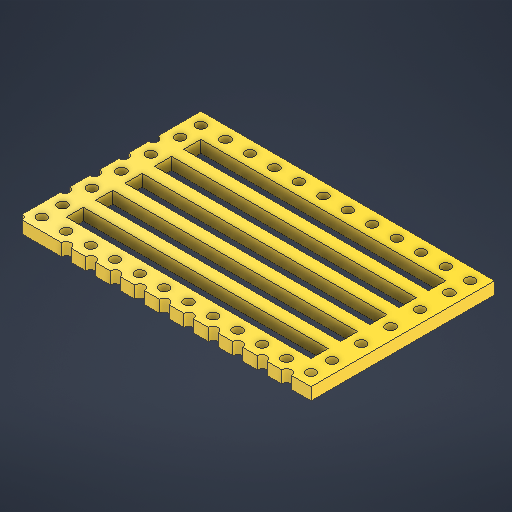
# Autodesk Inventor part: placa_galbena
Saved by Autodesk Inventor 2026.1 (Build 301233000, 233)
## iProperties
Created: 2025-09-04
Part Number: placa_galbena
Material: Generic
Document SubType Name: Modeling
Designer: emanuel
Density: 1 g/cm^3
Appearance: Default
Author: emanuel
Autodesk Inventor part; units mm, degrees
ref_plane "YZ Plane" through (0, 0, 0) normal (1, 0, 0) x (0, 1, 0)
ref_plane "XZ Plane" through (0, 0, 0) normal (0, 1, 0) x (-1, 0, 0)
ref_plane "XY Plane" through (0, 0, 0) normal (0, 0, 1) x (1, 0, 0)
sketch "Sketch1" plane through (0, 0, 0) normal (0, 1, 0) x (-1, 0, 0)
  line L0 (0, 0) -> (60, 0)
  line L1 (60, 0) -> (60, -37.5)
  line L2 (60, -37.5) -> (0, -37.5)
  line L3 (0, -37.5) -> (0, 0)
  line L4 (60, 0) -> (55, 0)
  line L5 (55, 0) -> (55, -5)
  line L6 (55, -5) -> (60, -5)
  line L7 (60, -5) -> (60, 0)
  line L8 (0, -37.5) -> (5, -37.5)
  line L9 (5, -37.5) -> (5, -32.5)
  line L10 (5, -32.5) -> (0, -32.5)
  line L11 (0, -32.5) -> (0, -37.5)
  line L12 (55, -5) -> (5, -5)
  line L13 (5, -5) -> (5, -32.5)
  line L14 (5, -32.5) -> (55, -32.5)
  line L15 (55, -32.5) -> (55, -5)
  line L16 (5, -5) -> (5, -8.5)
  line L17 (5, -8.5) -> (5, -11)
  line L18 (5, -11) -> (5, -14.5)
  line L19 (5, -14.5) -> (5, -17)
  line L20 (5, -17) -> (5, -20.5)
  line L21 (5, -20.5) -> (5, -23)
  line L22 (5, -23) -> (5, -26.5)
  line L23 (5, -26.5) -> (5, -29)
  line L24 (5, -29) -> (5, -32.5)
  line L25 (5, -8.5) -> (55, -8.5)
  line L26 (55, -8.5) -> (55, -11)
  line L27 (55, -11) -> (5, -11)
  line L28 (5, -11) -> (5, -8.5)
  line L29 (5, -14.5) -> (55, -14.5)
  line L30 (55, -14.5) -> (55, -17)
  line L31 (55, -17) -> (5, -17)
  line L32 (5, -17) -> (5, -14.5)
  line L33 (5, -20.5) -> (55, -20.5)
  line L34 (55, -20.5) -> (55, -23)
  line L35 (55, -23) -> (5, -23)
  line L36 (5, -23) -> (5, -20.5)
  line L37 (5, -26.5) -> (55, -26.5)
  line L38 (55, -26.5) -> (55, -29)
  line L39 (55, -29) -> (5, -29)
  line L40 (5, -29) -> (5, -26.5)
  line L41 (0, 0) -> (2.5, 0)
  line L42 (2.5, 0) -> (2.5, -2.5)
  line L43 (2.5, -2.5) -> (0, -2.5)
  line L44 (0, -2.5) -> (0, 0)
  circle A0 centre (2.5, -2.5) radius 1
  line L45 (5, -6.75) -> (2.5, -6.75)
  line L46 (5, -12.75) -> (2.5, -12.75)
  line L47 (5, -18.75) -> (2.5, -18.75)
  line L48 (5, -24.75) -> (2.5, -24.75)
  line L49 (5, -30.75) -> (2.5, -30.75)
  line L50 (5, -35) -> (2.5, -35)
  circle A1 centre (2.5, -35) radius 1
  circle A2 centre (2.5, -30.75) radius 1
  circle A3 centre (2.5, -24.75) radius 1
  circle A4 centre (2.5, -18.75) radius 1
  circle A5 centre (2.5, -12.75) radius 1
  circle A6 centre (2.5, -6.75) radius 1
  line L51 (60, 0) -> (57.5, 0)
  line L52 (57.5, 0) -> (57.5, -2.5)
  line L53 (57.5, -2.5) -> (60, -2.5)
  line L54 (60, -2.5) -> (60, 0)
  circle A7 centre (57.5, -2.5) radius 1
  circle A8 centre (57.5, -6.75) radius 1
  circle A9 centre (57.5, -12.75) radius 1
  circle A10 centre (57.5, -18.75) radius 1
  circle A11 centre (57.5, -24.75) radius 1
  circle A12 centre (57.5, -30.75) radius 1
  circle A13 centre (57.5, -35) radius 1
  line L55 (57.5, -35) -> (52.5, -35)
  line L56 (52.5, -35) -> (47.5, -35)
  line L57 (47.5, -35) -> (42.5, -35)
  line L58 (42.5, -35) -> (37.5, -35)
  line L59 (37.5, -35) -> (32.5, -35)
  line L60 (32.5, -35) -> (27.5, -35)
  line L61 (27.5, -35) -> (22.5, -35)
  line L62 (22.5, -35) -> (17.5, -35)
  line L63 (17.5, -35) -> (12.5, -35)
  line L64 (12.5, -35) -> (7.5, -35)
  circle A14 centre (52.5, -35) radius 1
  circle A15 centre (47.5, -35) radius 1
  circle A16 centre (42.5, -35) radius 1
  circle A17 centre (37.5, -35) radius 1
  circle A18 centre (32.5, -35) radius 1
  circle A19 centre (27.5, -35) radius 1
  circle A20 centre (22.5, -35) radius 1
  circle A21 centre (17.5, -35) radius 1
  circle A22 centre (12.5, -35) radius 1
  circle A23 centre (7.5, -35) radius 1
  circle A24 centre (52.5, -2.5) radius 1
  circle A25 centre (47.5, -2.5) radius 1
  circle A26 centre (42.5, -2.5) radius 1
  circle A27 centre (37.5, -2.5) radius 1
  circle A28 centre (32.5, -2.5) radius 1
  circle A29 centre (27.5, -2.5) radius 1
  circle A30 centre (22.5, -2.5) radius 1
  circle A31 centre (17.5, -2.5) radius 1
  circle A32 centre (12.5, -2.5) radius 1
  circle A33 centre (7.5, -2.5) radius 1
  line L65 (0, 0) -> (5, 0)
  line L66 (5, 0) -> (10, 0)
  line L67 (10, 0) -> (15, 0)
  line L68 (15, 0) -> (20, 0)
  line L69 (20, 0) -> (25, 0)
  line L70 (25, 0) -> (30, 0)
  line L71 (30, 0) -> (35, 0)
  line L72 (35, 0) -> (40, 0)
  line L73 (40, 0) -> (45, 0)
  line L74 (45, 0) -> (50, 0)
  line L75 (50, 0) -> (55, 0)
  circle A34 centre (5, 0) radius 1
  circle A35 centre (10, 0) radius 1
  circle A36 centre (15, 0) radius 1
  circle A37 centre (20, 0) radius 1
  circle A38 centre (25, 0) radius 1
  circle A39 centre (30, 0) radius 1
  circle A40 centre (35, 0) radius 1
  circle A41 centre (40, 0) radius 1
  circle A42 centre (45, 0) radius 1
  circle A43 centre (50, 0) radius 1
  circle A44 centre (60, 0) radius 1
  line L76 (55, -9.75) -> (60, -9.75)
  line L77 (55, -15.75) -> (60, -15.75)
  line L78 (55, -21.75) -> (60, -21.75)
  line L79 (55, -27.75) -> (60, -27.75)
  circle A45 centre (60, -27.75) radius 1
  circle A46 centre (60, -21.75) radius 1
  circle A47 centre (60, -15.75) radius 1
  circle A48 centre (60, -9.75) radius 1
  point P0 (60, -1)
  point P1 (59, 0)
  point P2 (51, 0)
  point P3 (49, 0)
  point P4 (46, 0)
  point P5 (44, 0)
  point P6 (41, 0)
  point P7 (39, 0)
  point P8 (36, 0)
  point P9 (34, 0)
  point P10 (31, 0)
  point P11 (29, 0)
  point P12 (26, 0)
  point P13 (24, 0)
  point P14 (21, 0)
  point P15 (19, 0)
  point P16 (16, 0)
  point P17 (14, 0)
  point P18 (11, 0)
  point P19 (9, 0)
  point P20 (6, 0)
  point P21 (4, 0)
  point P22 (60, -28.75)
  point P23 (60, -26.75)
  point P24 (60, -22.75)
  point P25 (60, -20.75)
  point P26 (60, -16.75)
  point P27 (60, -14.75)
  point P28 (60, -10.75)
  point P29 (60, -8.75)
  dimension "d0" = 60
  dimension "d1" = 37.5
  dimension "d2" = 5
  dimension "d3" = 5
  dimension "d4" = 5
  dimension "d5" = 5
  dimension "d6" = 3.5
  dimension "d7" = 2.5
  dimension "d8" = 3.5
  dimension "d9" = 2.5
  dimension "d10" = 3.5
  dimension "d11" = 2.5
  dimension "d12" = 3.5
  dimension "d13" = 2.5
  dimension "d14" = 3.5
  dimension "d15" = 2.5
  dimension "d16" = 2.5
  dimension "d17" = 2
  dimension "d18" = 2
  dimension "d19" = 2
  dimension "d20" = 2
  dimension "d21" = 2
  dimension "d22" = 2
  dimension "d23" = 2
  dimension "d24" = 2.5
  dimension "d25" = 2.5
  dimension "d26" = 2
  dimension "d27" = 2
  dimension "d28" = 2
  dimension "d29" = 2
  dimension "d30" = 2
  dimension "d31" = 2
  dimension "d32" = 2
  dimension "d33" = 5
  dimension "d34" = 5
  dimension "d35" = 5
  dimension "d36" = 5
  dimension "d37" = 5
  dimension "d38" = 5
  dimension "d39" = 5
  dimension "d40" = 5
  dimension "d41" = 5
  dimension "d42" = 5
  dimension "d43" = 2
  dimension "d44" = 2
  dimension "d45" = 2
  dimension "d46" = 2
  dimension "d47" = 2
  dimension "d48" = 2
  dimension "d49" = 2
  dimension "d50" = 2
  dimension "d51" = 2
  dimension "d52" = 2
  dimension "d53" = 2
  dimension "d54" = 2
  dimension "d55" = 2
  dimension "d56" = 2
  dimension "d57" = 2
  dimension "d58" = 2
  dimension "d59" = 2
  dimension "d60" = 2
  dimension "d61" = 2
  dimension "d62" = 2
  dimension "d63" = 5
  constraints: 156 end point, 49 centre point, 33 coincident, 20 parallel, 18 point on line, 17 horizontal, 11 perpendicular, 10 midpoint, 2 collinear, 2 vertical, 24 other
  measures "d0" distance of L1.end L2.end
  measures "d1" distance of L1.start L1.end
  measures "d2" distance of L6.end L5.end
  measures "d3" distance of L5.end L4.end
  measures "d4" distance of L10.end L9.end
  measures "d5" distance of L9.end L8.end
  measures "d6" distance of L12.end L16.end
  measures "d7" distance of L16.end L17.end
  measures "d8" distance of L17.end L18.end
  measures "d9" distance of L18.end L19.end
  measures "d10" distance of L19.end L20.end
  measures "d11" distance of L20.end L21.end
  measures "d12" distance of L21.end L22.end
  measures "d13" distance of L22.end L23.end
  measures "d14" distance of L23.end L9.end
  measures "d15" distance of L42.end L43.end
  measures "d16" distance of L41.end L42.end
  measures "d17" diameter of A0
  measures "d18" diameter of A1
  measures "d19" diameter of A2
  measures "d20" diameter of A3
  measures "d21" diameter of A4
  measures "d22" diameter of A5
  measures "d23" diameter of A6
  measures "d24" distance of L53.end L52.end
  measures "d25" distance of L52.end L51.end
  measures "d26" diameter of A7
  measures "d27" diameter of A8
  measures "d28" diameter of A9
  measures "d29" diameter of A10
  measures "d30" diameter of A11
  measures "d31" diameter of A12
  measures "d32" diameter of A13
  measures "d33" distance of L55.start L55.end
  measures "d34" distance of L55.end L56.end
  measures "d35" distance of L56.end L57.end
  measures "d36" distance of L57.end L58.end
  measures "d37" distance of L58.end L59.end
  measures "d38" distance of L59.end L60.end
  measures "d39" distance of L60.end L61.end
  measures "d40" distance of L61.end L62.end
  measures "d41" distance of L62.end L63.end
  measures "d42" distance of L63.end L64.end
  measures "d43" diameter of A14
  measures "d44" diameter of A15
  measures "d45" diameter of A16
  measures "d46" diameter of A17
  measures "d47" diameter of A18
  measures "d48" diameter of A19
  measures "d49" diameter of A20
  measures "d50" diameter of A21
  measures "d51" diameter of A22
  measures "d52" diameter of A23
  measures "d53" diameter of A24
  measures "d54" diameter of A25
  measures "d55" diameter of A26
  measures "d56" diameter of A27
  measures "d57" diameter of A28
  measures "d58" diameter of A29
  measures "d59" diameter of A30
  measures "d60" diameter of A31
  measures "d61" diameter of A32
  measures "d62" diameter of A33
  measures "d63" distance of L3.end L65.end
extrude "Extrusion1" add sketch "Sketch1" along normal blind 2.5 contours L0 L42 A0 L43 L3 | L0 A34 A35 A36 A37 A38 A39 A40 A41 A42 A43 L5 L12 L13 L10 L3 L43 A0 L42 | L10 L9 L2 L3 | L14 L15 L79 A45 L1 L2 L9 | L13 L37 L15 L39 | L15 L78 A46 L1 A45 L79 | L13 L33 L15 L35 | L15 L77 A47 L1 A46 L78 | L13 L29 L15 L31 | L15 L76 A48 L1 A47 L77 | L13 L25 L15 L27 | L15 L6 L1 A48 L76 | L5 L0 L52 A7 L53 L1 L6 | L53 A7 L52 L0 A44 L1
body "Solid1"
